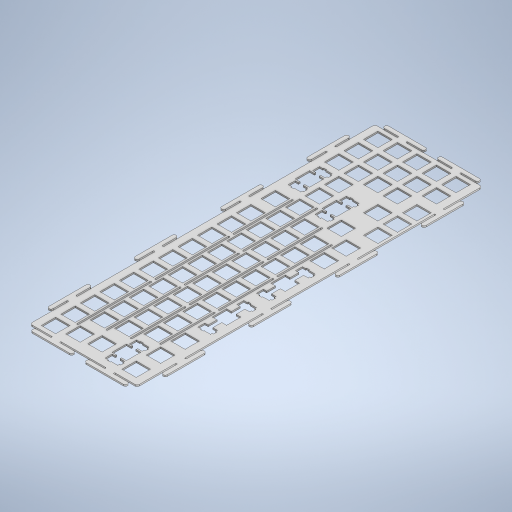
# Autodesk Inventor part: 定位板
Saved by Autodesk Inventor 2024 (Build 280153000, 153)
## iProperties
Created: 2023-06-19
Part Number: 定位板
Material: 常规
Document SubType Name: Modeling
Designer: 24564
Density: 1 g/cm^3
Appearance: 默认
Author: 24564
Autodesk Inventor part; units mm, degrees
(part 1 of 2)
ref_plane "YZ Plane" through (0, 0, 0) normal (1, 0, 0) x (0, 1, 0)
ref_plane "XZ Plane" through (0, 0, 0) normal (0, 1, 0) x (-1, 0, 0)
ref_plane "XY Plane" through (0, 0, 0) normal (0, 0, 1) x (1, 0, 0)
sketch "草图1" plane through (0, 0, 0) normal (0, 1, 0) x (-1, 0, 0)
  line L0 (104.4878, -334.8489) -> (0, -334.8489)
  line L1 (0, 1.4754) -> (104.4878, 1.4754)
  line L2 (16.5254, -235.8869) -> (16.5254, -249.8869)
  line L3 (16.5254, -249.8869) -> (2.5259, -249.8869)
  line L4 (2.5259, -235.8869) -> (16.5254, -235.8869)
  line L5 (16.5254, -254.9369) -> (16.5254, -268.9369)
  line L6 (16.5254, -268.9369) -> (2.5259, -268.9369)
  line L7 (2.5259, -254.9369) -> (16.5254, -254.9369)
  line L8 (16.5254, -273.9869) -> (16.5254, -287.9869)
  line L9 (16.5254, -287.9869) -> (2.5259, -287.9869)
  line L10 (2.5259, -273.9869) -> (16.5254, -273.9869)
  line L11 (21.2879, -93.0121) -> (16.5874, -93.0121)
  line L12 (16.5874, -93.0121) -> (16.5874, -84.3359)
  line L13 (16.5874, -84.3359) -> (19.8176, -84.3359)
  line L14 (19.8176, -84.3359) -> (19.8176, -77.5862)
  line L15 (19.8176, -77.5862) -> (16.5874, -77.5862)
  line L16 (16.5874, -77.5862) -> (16.5874, -76.7607)
  line L17 (16.5874, -76.7607) -> (13.7886, -76.7607)
  line L18 (13.7886, -76.7607) -> (13.7886, -77.5862)
  line L19 (13.7886, -77.5862) -> (7.5186, -77.5862)
  line L20 (7.5186, -77.5862) -> (7.5186, -79.3116)
  line L21 (7.5186, -79.3116) -> (6.3183, -79.3116)
  line L22 (6.3183, -79.3116) -> (6.3183, -82.6119)
  line L23 (6.3183, -82.6119) -> (7.5186, -82.6119)
  line L24 (7.5186, -82.6119) -> (7.5186, -84.3359)
  line L25 (7.5186, -84.3359) -> (11.9889, -84.3359)
  line L26 (11.9889, -84.3359) -> (11.9889, -93.0121)
  line L27 (11.9889, -93.0121) -> (7.2884, -93.0121)
  line L28 (7.2884, -93.0121) -> (7.2884, -107.0119)
  line L29 (7.2884, -107.0119) -> (11.9889, -107.0119)
  line L30 (11.9889, -107.0119) -> (11.9889, -115.6859)
  line L31 (11.9889, -115.6859) -> (7.5186, -115.6859)
  line L32 (7.5186, -115.6859) -> (7.5186, -117.4119)
  line L33 (7.5186, -117.4119) -> (6.3183, -117.4119)
  line L34 (6.3183, -117.4119) -> (6.3183, -120.7119)
  line L35 (6.3183, -120.7119) -> (7.5186, -120.7119)
  line L36 (7.5186, -120.7119) -> (7.5186, -122.4359)
  line L37 (7.5186, -122.4359) -> (13.7886, -122.4359)
  line L38 (13.7886, -122.4359) -> (13.7886, -123.2619)
  line L39 (13.7886, -123.2619) -> (16.5874, -123.2619)
  line L40 (16.5874, -123.2619) -> (16.5874, -122.4359)
  line L41 (16.5874, -122.4359) -> (19.8176, -122.4359)
  line L42 (19.8176, -122.4359) -> (19.8176, -115.6859)
  line L43 (19.8176, -115.6859) -> (16.5874, -115.6859)
  line L44 (16.5874, -115.6859) -> (16.5874, -107.0119)
  line L45 (16.5874, -107.0119) -> (21.2879, -107.0119)
  line L46 (21.2879, -107.0119) -> (21.2879, -93.0121)
  line L47 (21.2879, -150.1619) -> (16.5874, -150.1619)
  line L48 (16.5874, -150.1619) -> (16.5874, -141.4859)
  line L49 (16.5874, -141.4859) -> (19.8176, -141.4859)
  line L50 (19.8176, -141.4859) -> (19.8176, -134.7359)
  line L51 (19.8176, -134.7359) -> (16.5874, -134.7359)
  line L52 (16.5874, -134.7359) -> (16.5874, -133.9109)
  line L53 (16.5874, -133.9109) -> (13.7886, -133.9109)
  line L54 (13.7886, -133.9109) -> (13.7886, -134.7359)
  line L55 (13.7886, -134.7359) -> (7.5186, -134.7359)
  line L56 (7.5186, -134.7359) -> (7.5186, -136.4619)
  line L57 (7.5186, -136.4619) -> (6.3183, -136.4619)
  line L58 (6.3183, -136.4619) -> (6.3183, -139.7619)
  line L59 (6.3183, -139.7619) -> (7.5186, -139.7619)
  line L60 (7.5186, -139.7619) -> (7.5186, -141.4859)
  line L61 (7.5186, -141.4859) -> (11.9889, -141.4859)
  line L62 (11.9889, -141.4859) -> (11.9889, -150.1619)
  line L63 (11.9889, -150.1619) -> (7.2884, -150.1619)
  line L64 (7.2884, -150.1619) -> (7.2884, -164.1619)
  line L65 (7.2884, -164.1619) -> (11.9889, -164.1619)
  line L66 (11.9889, -164.1619) -> (11.9889, -172.8359)
  line L67 (11.9889, -172.8359) -> (7.5186, -172.8359)
  line L68 (7.5186, -172.8359) -> (7.5186, -174.5619)
  line L69 (7.5186, -174.5619) -> (6.3183, -174.5619)
  line L70 (6.3183, -174.5619) -> (6.3183, -177.8619)
  line L71 (6.3183, -177.8619) -> (7.5186, -177.8619)
  line L72 (7.5186, -177.8619) -> (7.5186, -179.5859)
  line L73 (7.5186, -179.5859) -> (13.7886, -179.5859)
  line L74 (13.7886, -179.5859) -> (13.7886, -180.4119)
  line L75 (13.7886, -180.4119) -> (16.5874, -180.4119)
  line L76 (16.5874, -180.4119) -> (16.5874, -179.5859)
  line L77 (16.5874, -179.5859) -> (19.8176, -179.5859)
  line L78 (19.8176, -179.5859) -> (19.8176, -172.8359)
  line L79 (19.8176, -172.8359) -> (16.5874, -172.8359)
  line L80 (16.5874, -172.8359) -> (16.5874, -164.1619)
  line L81 (16.5874, -164.1619) -> (21.2879, -164.1619)
  line L82 (21.2879, -164.1619) -> (21.2879, -150.1619)
  line L83 (21.2879, -4.9058) -> (21.2879, -18.9053)
  line L84 (21.2879, -18.9053) -> (7.2884, -18.9053)
  line L85 (7.2884, -18.9053) -> (7.2884, -4.9058)
  line L86 (7.2884, -4.9058) -> (21.2879, -4.9058)
  line L87 (21.2879, -28.7169) -> (21.2879, -42.7177)
  line L88 (21.2879, -42.7177) -> (7.2884, -42.7177)
  line L89 (7.2884, -42.7177) -> (7.2884, -28.7169)
  line L90 (7.2884, -28.7169) -> (21.2879, -28.7169)
  line L91 (21.2879, -52.5309) -> (21.2879, -66.5302)
  line L92 (21.2879, -66.5302) -> (7.2884, -66.5302)
  line L93 (7.2884, -66.5302) -> (7.2884, -52.5309)
  line L94 (7.2884, -52.5309) -> (21.2879, -52.5309)
  line L95 (21.2879, -188.2619) -> (21.2879, -202.2619)
  line L96 (21.2879, -202.2619) -> (7.2884, -202.2619)
  line L97 (7.2884, -202.2619) -> (7.2884, -188.2619)
  line L98 (7.2884, -188.2619) -> (21.2879, -188.2619)
  line L99 (21.2879, -209.6919) -> (21.2879, -223.6929)
  line L100 (21.2879, -223.6929) -> (7.2884, -223.6929)
  line L101 (7.2884, -223.6929) -> (7.2884, -209.6919)
  line L102 (7.2884, -209.6919) -> (21.2879, -209.6919)
  line L103 (21.2879, -297.7999) -> (21.2879, -311.7989)
  line L104 (21.2879, -311.7989) -> (7.2884, -311.7989)
  line L105 (7.2884, -311.7989) -> (7.2884, -297.7999)
  line L106 (7.2884, -297.7999) -> (21.2879, -297.7999)
  line L107 (21.2879, -316.8499) -> (21.2879, -330.8489)
  line L108 (21.2879, -330.8489) -> (7.2884, -330.8489)
  line L109 (7.2884, -330.8489) -> (7.2884, -316.8499)
  line L110 (7.2884, -316.8499) -> (21.2879, -316.8499)
  line L111 (35.5753, -254.9369) -> (35.5753, -268.9369)
  line L112 (35.5753, -268.9369) -> (21.5759, -268.9369)
  line L113 (21.5759, -268.9369) -> (21.5759, -254.9369)
  line L114 (21.5759, -254.9369) -> (35.5753, -254.9369)
  line L115 (40.3378, -14.4308) -> (35.6374, -14.4308)
  line L116 (35.6374, -14.4308) -> (35.6374, -12.9053)
  line L117 (35.6374, -12.9053) -> (38.8675, -12.9053)
  line L118 (38.8675, -12.9053) -> (38.8675, -6.1557)
  line L119 (38.8675, -6.1557) -> (35.6374, -6.1557)
  line L120 (35.6374, -6.1557) -> (35.6374, -5.3302)
  line L121 (35.6374, -5.3302) -> (32.8386, -5.3302)
  line L122 (32.8386, -5.3302) -> (32.8386, -6.1557)
  line L123 (32.8386, -6.1557) -> (26.5686, -6.1557)
  line L124 (26.5686, -6.1557) -> (26.5686, -7.881)
  line L125 (26.5686, -7.881) -> (25.3683, -7.881)
  line L126 (25.3683, -7.881) -> (25.3683, -11.18)
  line L127 (25.3683, -11.18) -> (26.5686, -11.18)
  line L128 (26.5686, -11.18) -> (26.5686, -12.9053)
  line L129 (26.5686, -12.9053) -> (31.0375, -12.9053)
  line L130 (31.0375, -12.9053) -> (31.0375, -14.4308)
  line L131 (31.0375, -14.4308) -> (26.3384, -14.4308)
  line L132 (26.3384, -14.4308) -> (26.3384, -28.4303)
  line L133 (26.3384, -28.4303) -> (31.0375, -28.4303)
  line L134 (31.0375, -28.4303) -> (31.0375, -29.9558)
  line L135 (31.0375, -29.9558) -> (26.5686, -29.9558)
  line L136 (26.5686, -29.9558) -> (26.5686, -31.6797)
  line L137 (26.5686, -31.6797) -> (25.3683, -31.6797)
  line L138 (25.3683, -31.6797) -> (25.3683, -34.9801)
  line L139 (25.3683, -34.9801) -> (26.5686, -34.9801)
  line L140 (26.5686, -34.9801) -> (26.5686, -36.7053)
  line L141 (26.5686, -36.7053) -> (32.8386, -36.7053)
  line L142 (32.8386, -36.7053) -> (32.8386, -37.5308)
  line L143 (32.8386, -37.5308) -> (35.6374, -37.5308)
  line L144 (35.6374, -37.5308) -> (35.6374, -36.7053)
  line L145 (35.6374, -36.7053) -> (38.8675, -36.7053)
  line L146 (38.8675, -36.7053) -> (38.8675, -29.9558)
  line L147 (38.8675, -29.9558) -> (35.6374, -29.9558)
  line L148 (35.6374, -29.9558) -> (35.6374, -28.4303)
  line L149 (35.6374, -28.4303) -> (40.3378, -28.4303)
  line L150 (40.3378, -28.4303) -> (40.3378, -14.4308)
  line L151 (40.3378, -45.3871) -> (40.3378, -59.3864)
  line L152 (40.3378, -59.3864) -> (26.3384, -59.3864)
  line L153 (26.3384, -59.3864) -> (26.3384, -45.3871)
  line L154 (26.3384, -45.3871) -> (40.3378, -45.3871)
  line L155 (40.3378, -64.4371) -> (40.3378, -78.4364)
  line L156 (40.3378, -78.4364) -> (26.3384, -78.4364)
  line L157 (26.3384, -78.4364) -> (26.3384, -64.4371)
  line L158 (26.3384, -64.4371) -> (40.3378, -64.4371)
  line L159 (40.3378, -83.4871) -> (40.3378, -97.4864)
  line L160 (40.3378, -97.4864) -> (26.3384, -97.4864)
  line L161 (26.3384, -97.4864) -> (26.3384, -83.4871)
  line L162 (26.3384, -83.4871) -> (40.3378, -83.4871)
  line L163 (40.3378, -102.5369) -> (40.3378, -116.5369)
  line L164 (40.3378, -116.5369) -> (26.3384, -116.5369)
  line L165 (26.3384, -116.5369) -> (26.3384, -102.5369)
  line L166 (26.3384, -102.5369) -> (40.3378, -102.5369)
  line L167 (40.3378, -121.5869) -> (40.3378, -135.5869)
  line L168 (40.3378, -135.5869) -> (26.3384, -135.5869)
  line L169 (26.3384, -135.5869) -> (26.3384, -121.5869)
  line L170 (26.3384, -121.5869) -> (40.3378, -121.5869)
  line L171 (40.3378, -140.6369) -> (40.3378, -154.6369)
  line L172 (40.3378, -154.6369) -> (26.3384, -154.6369)
  line L173 (26.3384, -154.6369) -> (26.3384, -140.6369)
  line L174 (26.3384, -140.6369) -> (40.3378, -140.6369)
  line L175 (40.3378, -159.6869) -> (40.3378, -173.6869)
  line L176 (40.3378, -173.6869) -> (26.3384, -173.6869)
  line L177 (26.3384, -173.6869) -> (26.3384, -159.6869)
  line L178 (26.3384, -159.6869) -> (40.3378, -159.6869)
  line L179 (40.3378, -178.7369) -> (40.3378, -192.7369)
  line L180 (40.3378, -192.7369) -> (26.3384, -192.7369)
  line L181 (26.3384, -192.7369) -> (26.3384, -178.7369)
  line L182 (26.3384, -178.7369) -> (40.3378, -178.7369)
  line L183 (40.3378, -197.7869) -> (40.3378, -211.7869)
  line L184 (40.3378, -211.7869) -> (26.3384, -211.7869)
  line L185 (26.3384, -211.7869) -> (26.3384, -197.7869)
  line L186 (26.3384, -197.7869) -> (40.3378, -197.7869)
  line L187 (40.3378, -223.9809) -> (40.3378, -237.9799)
  line L188 (40.3378, -237.9799) -> (26.3384, -237.9799)
  line L189 (26.3384, -237.9799) -> (26.3384, -223.9809)
  line L190 (26.3384, -223.9809) -> (40.3378, -223.9809)
  line L191 (40.3378, -278.7499) -> (40.3378, -292.7489)
  line L192 (40.3378, -292.7489) -> (26.3384, -292.7489)
  line L193 (26.3384, -292.7489) -> (26.3384, -278.7499)
  line L194 (26.3384, -278.7499) -> (40.3378, -278.7499)
  line L195 (40.3378, -297.7999) -> (40.3378, -311.7989)
  line L196 (40.3378, -311.7989) -> (26.3384, -311.7989)
  line L197 (26.3384, -311.7989) -> (26.3384, -297.7999)
  line L198 (26.3384, -297.7999) -> (40.3378, -297.7999)
  line L199 (40.3378, -316.8499) -> (40.3378, -330.8489)
  line L200 (40.3378, -330.8489) -> (26.3384, -330.8489)
  line L201 (26.3384, -330.8489) -> (26.3384, -316.8499)
  line L202 (26.3384, -316.8499) -> (40.3378, -316.8499)
  line L203 (59.3878, -238.2669) -> (54.6874, -238.2669)
  line L204 (54.6874, -238.2669) -> (54.6874, -236.7429)
  line L205 (54.6874, -236.7429) -> (57.9175, -236.7429)
  line L206 (57.9175, -236.7429) -> (57.9175, -229.9919)
  line L207 (57.9175, -229.9919) -> (54.6874, -229.9919)
  line L208 (54.6874, -229.9919) -> (54.6874, -229.1679)
  line L209 (54.6874, -229.1679) -> (51.8885, -229.1679)
  line L210 (51.8885, -229.1679) -> (51.8885, -229.9919)
  line L211 (51.8885, -229.9919) -> (45.6186, -229.9919)
  line L212 (45.6186, -229.9919) -> (45.6186, -231.7169)
  line L213 (45.6186, -231.7169) -> (44.4184, -231.7169)
  line L214 (44.4184, -231.7169) -> (44.4184, -235.0179)
  line L215 (44.4184, -235.0179) -> (45.6186, -235.0179)
  line L216 (45.6186, -235.0179) -> (45.6186, -236.7429)
  line L217 (45.6186, -236.7429) -> (50.0876, -236.7429)
  line L218 (50.0876, -236.7429) -> (50.0876, -238.2669)
  line L219 (50.0876, -238.2669) -> (45.3886, -238.2669)
  line L220 (45.3886, -238.2669) -> (45.3886, -252.2659)
  line L221 (45.3886, -252.2659) -> (50.0876, -252.2659)
  line L222 (50.0876, -252.2659) -> (50.0876, -253.7919)
  line L223 (50.0876, -253.7919) -> (45.6186, -253.7919)
  line L224 (45.6186, -253.7919) -> (45.6186, -255.5159)
  line L225 (45.6186, -255.5159) -> (44.4184, -255.5159)
  line L226 (44.4184, -255.5159) -> (44.4184, -258.8179)
  line L227 (44.4184, -258.8179) -> (45.6186, -258.8179)
  line L228 (45.6186, -258.8179) -> (45.6186, -260.5429)
  line L229 (45.6186, -260.5429) -> (51.8885, -260.5429)
  line L230 (51.8885, -260.5429) -> (51.8885, -261.3669)
  line L231 (51.8885, -261.3669) -> (54.6874, -261.3669)
  line L232 (54.6874, -261.3669) -> (54.6874, -260.5429)
  line L233 (54.6874, -260.5429) -> (57.9175, -260.5429)
  line L234 (57.9175, -260.5429) -> (57.9175, -253.7919)
  line L235 (57.9175, -253.7919) -> (54.6874, -253.7919)
  line L236 (54.6874, -253.7919) -> (54.6874, -252.2659)
  line L237 (54.6874, -252.2659) -> (59.3878, -252.2659)
  line L238 (59.3878, -252.2659) -> (59.3878, -238.2669)
  line L239 (59.3878, -9.6669) -> (59.3878, -23.6678)
  line L240 (59.3878, -23.6678) -> (45.3886, -23.6678)
  line L241 (45.3886, -23.6678) -> (45.3886, -9.6669)
  line L242 (45.3886, -9.6669) -> (59.3878, -9.6669)
  line L243 (59.3878, -35.8621) -> (59.3878, -49.8614)
  line L244 (59.3878, -49.8614) -> (45.3886, -49.8614)
  line L245 (45.3886, -49.8614) -> (45.3886, -35.8621)
  line L246 (45.3886, -35.8621) -> (59.3878, -35.8621)
  line L247 (59.3878, -54.9121) -> (59.3878, -68.9114)
  line L248 (59.3878, -68.9114) -> (45.3886, -68.9114)
  line L249 (45.3886, -68.9114) -> (45.3886, -54.9121)
  line L250 (45.3886, -54.9121) -> (59.3878, -54.9121)
  line L251 (59.3878, -73.9621) -> (59.3878, -87.9614)
  line L252 (59.3878, -87.9614) -> (45.3886, -87.9614)
  line L253 (45.3886, -87.9614) -> (45.3886, -73.9621)
  line L254 (45.3886, -73.9621) -> (59.3878, -73.9621)
  line L255 (59.3878, -93.0121) -> (59.3878, -107.0119)
  line L256 (59.3878, -107.0119) -> (45.3886, -107.0119)
  line L257 (45.3886, -107.0119) -> (45.3886, -93.0121)
  line L258 (45.3886, -93.0121) -> (59.3878, -93.0121)
  line L259 (59.3878, -112.0619) -> (59.3878, -126.0619)
  line L260 (59.3878, -126.0619) -> (45.3886, -126.0619)
  line L261 (45.3886, -126.0619) -> (45.3886, -112.0619)
  line L262 (45.3886, -112.0619) -> (59.3878, -112.0619)
  line L263 (59.3878, -131.1119) -> (59.3878, -145.1119)
  line L264 (59.3878, -145.1119) -> (45.3886, -145.1119)
  line L265 (45.3886, -145.1119) -> (45.3886, -131.1119)
  line L266 (45.3886, -131.1119) -> (59.3878, -131.1119)
  line L267 (59.3878, -150.1619) -> (59.3878, -164.1619)
  line L268 (59.3878, -164.1619) -> (45.3886, -164.1619)
  line L269 (45.3886, -164.1619) -> (45.3886, -150.1619)
  line L270 (45.3886, -150.1619) -> (59.3878, -150.1619)
  line L271 (59.3878, -169.2119) -> (59.3878, -183.2119)
  line L272 (59.3878, -183.2119) -> (45.3886, -183.2119)
  line L273 (45.3886, -183.2119) -> (45.3886, -169.2119)
  line L274 (45.3886, -169.2119) -> (59.3878, -169.2119)
  line L275 (59.3878, -188.2619) -> (59.3878, -202.2619)
  line L276 (59.3878, -202.2619) -> (45.3886, -202.2619)
  line L277 (45.3886, -202.2619) -> (45.3886, -188.2619)
  line L278 (45.3886, -188.2619) -> (59.3878, -188.2619)
  line L279 (59.3878, -207.3119) -> (59.3878, -221.3119)
  line L280 (59.3878, -221.3119) -> (45.3886, -221.3119)
  line L281 (45.3886, -221.3119) -> (45.3886, -207.3119)
  line L282 (45.3886, -207.3119) -> (59.3878, -207.3119)
  line L283 (59.3878, -278.7499) -> (59.3878, -292.7489)
  line L284 (59.3878, -292.7489) -> (45.3886, -292.7489)
  line L285 (45.3886, -292.7489) -> (45.3886, -278.7499)
  line L286 (45.3886, -278.7499) -> (59.3878, -278.7499)
  line L287 (59.3878, -297.7999) -> (59.3878, -311.7989)
  line L288 (59.3878, -311.7989) -> (45.3886, -311.7989)
  line L289 (45.3886, -311.7989) -> (45.3886, -297.7999)
  line L290 (45.3886, -297.7999) -> (59.3878, -297.7999)
  line L291 (59.3878, -316.8499) -> (59.3878, -330.8489)
  line L292 (59.3878, -330.8489) -> (45.3886, -330.8489)
  line L293 (45.3886, -330.8489) -> (45.3886, -316.8499)
  line L294 (45.3886, -316.8499) -> (59.3878, -316.8499)
  line L295 (78.4378, -7.2871) -> (78.4378, -21.2866)
  line L296 (78.4378, -21.2866) -> (64.4386, -21.2866)
  line L297 (64.4386, -21.2866) -> (64.4386, -7.2871)
  line L298 (64.4386, -7.2871) -> (78.4378, -7.2871)
  line L299 (78.4378, -31.0996) -> (78.4378, -45.0989)
  line L300 (78.4378, -45.0989) -> (64.4386, -45.0989)
  line L301 (64.4386, -45.0989) -> (64.4386, -31.0996)
  line L302 (64.4386, -31.0996) -> (78.4378, -31.0996)
  line L303 (78.4378, -50.1496) -> (78.4378, -64.1489)
  line L304 (78.4378, -64.1489) -> (64.4386, -64.1489)
  line L305 (64.4386, -64.1489) -> (64.4386, -50.1496)
  line L306 (64.4386, -50.1496) -> (78.4378, -50.1496)
  line L307 (78.4378, -69.1996) -> (78.4378, -83.1989)
  line L308 (78.4378, -83.1989) -> (64.4386, -83.1989)
  line L309 (64.4386, -83.1989) -> (64.4386, -69.1996)
  line L310 (64.4386, -69.1996) -> (78.4378, -69.1996)
  line L311 (78.4378, -88.2496) -> (78.4378, -102.2489)
  line L312 (78.4378, -102.2489) -> (64.4386, -102.2489)
  line L313 (64.4386, -102.2489) -> (64.4386, -88.2496)
  line L314 (64.4386, -88.2496) -> (78.4378, -88.2496)
  line L315 (78.4378, -107.2999) -> (78.4378, -121.2989)
  line L316 (78.4378, -121.2989) -> (64.4386, -121.2989)
  line L317 (64.4386, -121.2989) -> (64.4386, -107.2999)
  line L318 (64.4386, -107.2999) -> (78.4378, -107.2999)
  line L319 (78.4378, -126.3499) -> (78.4378, -140.3489)
  line L320 (78.4378, -140.3489) -> (64.4386, -140.3489)
  line L321 (64.4386, -140.3489) -> (64.4386, -126.3499)
  line L322 (64.4386, -126.3499) -> (78.4378, -126.3499)
  line L323 (78.4378, -145.3999) -> (78.4378, -159.3989)
  line L324 (78.4378, -159.3989) -> (64.4386, -159.3989)
  line L325 (64.4386, -159.3989) -> (64.4386, -145.3999)
  line L326 (64.4386, -145.3999) -> (78.4378, -145.3999)
  line L327 (78.4378, -164.4499) -> (78.4378, -178.4489)
  line L328 (78.4378, -178.4489) -> (64.4386, -178.4489)
  line L329 (64.4386, -178.4489) -> (64.4386, -164.4499)
  line L330 (64.4386, -164.4499) -> (78.4378, -164.4499)
  line L331 (78.4378, -183.4999) -> (78.4378, -197.4989)
  line L332 (78.4378, -197.4989) -> (64.4386, -197.4989)
  line L333 (64.4386, -197.4989) -> (64.4386, -183.4999)
  line L334 (64.4386, -183.4999) -> (78.4378, -183.4999)
  line L335 (78.4378, -202.5499) -> (78.4378, -216.5489)
  line L336 (78.4378, -216.5489) -> (64.4386, -216.5489)
  line L337 (64.4386, -216.5489) -> (64.4386, -202.5499)
  line L338 (64.4386, -202.5499) -> (78.4378, -202.5499)
  line L339 (78.4378, -221.5999) -> (78.4378, -235.5989)
  line L340 (78.4378, -235.5989) -> (64.4386, -235.5989)
  line L341 (64.4386, -235.5989) -> (64.4386, -221.5999)
  line L342 (64.4386, -221.5999) -> (78.4378, -221.5999)
  line L343 (78.4378, -240.6499) -> (78.4378, -254.6489)
  line L344 (78.4378, -254.6489) -> (64.4386, -254.6489)
  line L345 (64.4386, -254.6489) -> (64.4386, -240.6499)
  line L346 (64.4386, -240.6499) -> (78.4378, -240.6499)
  line L347 (78.4378, -259.6999) -> (78.4378, -273.6989)
  line L348 (78.4378, -273.6989) -> (64.4386, -273.6989)
  line L349 (64.4386, -273.6989) -> (64.4386, -259.6999)
  line L350 (64.4386, -259.6999) -> (78.4378, -259.6999)
  line L351 (78.4378, -278.7499) -> (78.4378, -292.7489)
  line L352 (78.4378, -292.7489) -> (64.4386, -292.7489)
  line L353 (64.4386, -292.7489) -> (64.4386, -278.7499)
  line L354 (64.4386, -278.7499) -> (78.4378, -278.7499)
  line L355 (78.4378, -297.7999) -> (78.4378, -311.7989)
  line L356 (78.4378, -311.7989) -> (64.4386, -311.7989)
  line L357 (64.4386, -311.7989) -> (64.4386, -297.7999)
  line L358 (64.4386, -297.7999) -> (78.4378, -297.7999)
  line L359 (78.4378, -316.8499) -> (78.4378, -330.8489)
  line L360 (78.4378, -330.8489) -> (64.4386, -330.8489)
  line L361 (64.4386, -330.8489) -> (64.4386, -316.8499)
  line L362 (64.4386, -316.8499) -> (78.4378, -316.8499)
  line L363 (97.4878, -250.1749) -> (92.7874, -250.1749)
  line L364 (92.7874, -250.1749) -> (92.7874, -248.6489)
  line L365 (92.7874, -248.6489) -> (96.0175, -248.6489)
  line L366 (96.0175, -248.6489) -> (96.0175, -241.8999)
  line L367 (96.0175, -241.8999) -> (92.7874, -241.8999)
  line L368 (92.7874, -241.8999) -> (92.7874, -241.0739)
  line L369 (92.7874, -241.0739) -> (89.9885, -241.0739)
  line L370 (89.9885, -241.0739) -> (89.9885, -241.8999)
  line L371 (89.9885, -241.8999) -> (83.7186, -241.8999)
  line L372 (83.7186, -241.8999) -> (83.7186, -243.6249)
  line L373 (83.7186, -243.6249) -> (82.5184, -243.6249)
  line L374 (82.5184, -243.6249) -> (82.5184, -246.9239)
  line L375 (82.5184, -246.9239) -> (83.7186, -246.9239)
  line L376 (83.7186, -246.9239) -> (83.7186, -248.6489)
  line L377 (83.7186, -248.6489) -> (88.1876, -248.6489)
  line L378 (88.1876, -248.6489) -> (88.1876, -250.1749)
  line L379 (88.1876, -250.1749) -> (83.4886, -250.1749)
  line L380 (83.4886, -250.1749) -> (83.4886, -264.1739)
  line L381 (83.4886, -264.1739) -> (88.1876, -264.1739)
  line L382 (88.1876, -264.1739) -> (88.1876, -265.6999)
  line L383 (88.1876, -265.6999) -> (83.7186, -265.6999)
  line L384 (83.7186, -265.6999) -> (83.7186, -267.4249)
  line L385 (83.7186, -267.4249) -> (82.5184, -267.4249)
  line L386 (82.5184, -267.4249) -> (82.5184, -270.7239)
  line L387 (82.5184, -270.7239) -> (83.7186, -270.7239)
  line L388 (83.7186, -270.7239) -> (83.7186, -272.4489)
  line L389 (83.7186, -272.4489) -> (89.9885, -272.4489)
  line L390 (89.9885, -272.4489) -> (89.9885, -273.2749)
  line L391 (89.9885, -273.2749) -> (92.7874, -273.2749)
  line L392 (92.7874, -273.2749) -> (92.7874, -272.4489)
  line L393 (92.7874, -272.4489) -> (96.0175, -272.4489)
  line L394 (96.0175, -272.4489) -> (96.0175, -265.6999)
  line L395 (96.0175, -265.6999) -> (92.7874, -265.6999)
  line L396 (92.7874, -265.6999) -> (92.7874, -264.1739)
  line L397 (92.7874, -264.1739) -> (97.4878, -264.1739)
  line L398 (97.4878, -264.1739) -> (97.4878, -250.1749)
  line L399 (97.4878, -2.5246) -> (97.4878, -16.5241)
  line L400 (97.4878, -16.5241) -> (83.4886, -16.5241)
  line L401 (83.4886, -16.5241) -> (83.4886, -2.5246)
  line L402 (83.4886, -2.5246) -> (97.4878, -2.5246)
  line L403 (97.4878, -21.5746) -> (97.4878, -35.5739)
  line L404 (97.4878, -35.5739) -> (83.4886, -35.5739)
  line L405 (83.4886, -35.5739) -> (83.4886, -21.5746)
  line L406 (83.4886, -21.5746) -> (97.4878, -21.5746)
  line L407 (97.4878, -40.6246) -> (97.4878, -54.6239)
  line L408 (97.4878, -54.6239) -> (83.4886, -54.6239)
  line L409 (83.4886, -54.6239) -> (83.4886, -40.6246)
  line L410 (83.4886, -40.6246) -> (97.4878, -40.6246)
  line L411 (97.4878, -59.6746) -> (97.4878, -73.6739)
  line L412 (97.4878, -73.6739) -> (83.4886, -73.6739)
  line L413 (83.4886, -73.6739) -> (83.4886, -59.6746)
  line L414 (83.4886, -59.6746) -> (97.4878, -59.6746)
  line L415 (97.4878, -78.7246) -> (97.4878, -92.7239)
  line L416 (97.4878, -92.7239) -> (83.4886, -92.7239)
  line L417 (83.4886, -92.7239) -> (83.4886, -78.7246)
  line L418 (83.4886, -78.7246) -> (97.4878, -78.7246)
  line L419 (97.4878, -97.7732) -> (97.4878, -111.7739)
  line L420 (97.4878, -111.7739) -> (83.4886, -111.7739)
  line L421 (83.4886, -111.7739) -> (83.4886, -97.7732)
  line L422 (83.4886, -97.7732) -> (97.4878, -97.7732)
  line L423 (97.4878, -116.8229) -> (97.4878, -130.8239)
  line L424 (97.4878, -130.8239) -> (83.4886, -130.8239)
  line L425 (83.4886, -130.8239) -> (83.4886, -116.8229)
  line L426 (83.4886, -116.8229) -> (97.4878, -116.8229)
  line L427 (97.4878, -135.8749) -> (97.4878, -149.8739)
  line L428 (97.4878, -149.8739) -> (83.4886, -149.8739)
  line L429 (83.4886, -149.8739) -> (83.4886, -135.8749)
  line L430 (83.4886, -135.8749) -> (97.4878, -135.8749)
  line L431 (97.4878, -154.9249) -> (97.4878, -168.9239)
  line L432 (97.4878, -168.9239) -> (83.4886, -168.9239)
  line L433 (83.4886, -168.9239) -> (83.4886, -154.9249)
  line L434 (83.4886, -154.9249) -> (97.4878, -154.9249)
  line L435 (97.4878, -173.9749) -> (97.4878, -187.9739)
  line L436 (97.4878, -187.9739) -> (83.4886, -187.9739)
  line L437 (83.4886, -187.9739) -> (83.4886, -173.9749)
  line L438 (83.4886, -173.9749) -> (97.4878, -173.9749)
  line L439 (97.4878, -193.0249) -> (97.4878, -207.0239)
  line L440 (97.4878, -207.0239) -> (83.4886, -207.0239)
  line L441 (83.4886, -207.0239) -> (83.4886, -193.0249)
  line L442 (83.4886, -193.0249) -> (97.4878, -193.0249)
  line L443 (97.4878, -216.8369) -> (97.4878, -230.8369)
  line L444 (97.4878, -230.8369) -> (83.4886, -230.8369)
  line L445 (83.4886, -230.8369) -> (83.4886, -216.8369)
  line L446 (83.4886, -216.8369) -> (97.4878, -216.8369)
  line L447 (97.4878, -278.7499) -> (97.4878, -292.7489)
  line L448 (97.4878, -292.7489) -> (83.4886, -292.7489)
  line L449 (83.4886, -292.7489) -> (83.4886, -278.7499)
  line L450 (83.4886, -278.7499) -> (97.4878, -278.7499)
  line L451 (97.4878, -297.7999) -> (97.4878, -311.7989)
  line L452 (97.4878, -311.7989) -> (83.4886, -311.7989)
  line L453 (83.4886, -311.7989) -> (83.4886, -297.7999)
  line L454 (83.4886, -297.7999) -> (97.4878, -297.7999)
  line L455 (97.4878, -316.8499) -> (97.4878, -330.8489)
  line L456 (97.4878, -330.8489) -> (83.4886, -330.8489)
  line L457 (83.4886, -330.8489) -> (83.4886, -316.8499)
  line L458 (83.4886, -316.8499) -> (97.4878, -316.8499)
  line L459 (81.7132, -21.5746) -> (81.7132, -92.7239)
  line L460 (80.2132, -92.7239) -> (80.2132, -21.5746)
  arc A0 (81.7132, -21.5746) -> (80.2132, -21.5746) centre (80.9632, -21.5746) ccw
  arc A1 (80.2132, -92.7239) -> (81.7132, -92.7239) centre (80.9632, -92.7239) ccw
  line L461 (62.6632, -31.0996) -> (62.6632, -102.2489)
  line L462 (61.1632, -102.2489) -> (61.1632, -31.0996)
  arc A2 (62.6632, -31.0996) -> (61.1632, -31.0996) centre (61.9132, -31.0996) ccw
  arc A3 (61.1632, -102.2489) -> (62.6632, -102.2489) centre (61.9132, -102.2489) ccw
  line L463 (62.6632, -107.2999) -> (62.6632, -159.3989)
  line L464 (61.1632, -159.3989) -> (61.1632, -107.2999)
  arc A4 (62.6632, -107.2999) -> (61.1632, -107.2999) centre (61.9132, -107.2999) ccw
  arc A5 (61.1632, -159.3989) -> (62.6632, -159.3989) centre (61.9132, -159.3989) ccw
  line L465 (43.6132, -35.8621) -> (43.6132, -87.9611)
  line L466 (42.1132, -87.9611) -> (42.1132, -35.8621)
  arc A6 (43.6132, -35.8621) -> (42.1132, -35.8621) centre (42.8632, -35.8621) ccw
  arc A7 (42.1132, -87.9611) -> (43.6132, -87.9611) centre (42.8632, -87.9611) ccw
  line L467 (24.5632, -45.3871) -> (24.5632, -97.4861)
  line L468 (23.0632, -97.4861) -> (23.0632, -45.3871)
  arc A8 (24.5632, -45.3871) -> (23.0632, -45.3871) centre (23.8132, -45.3871) ccw
  arc A9 (23.0632, -97.4861) -> (24.5632, -97.4861) centre (23.8132, -97.4861) ccw
  line L469 (24.5632, -102.5369) -> (24.5632, -154.6359)
  line L470 (23.0632, -154.6359) -> (23.0632, -102.5369)
  arc A10 (24.5632, -102.5369) -> (23.0632, -102.5369) centre (23.8132, -102.5369) ccw
  arc A11 (23.0632, -154.6359) -> (24.5632, -154.6359) centre (23.8132, -154.6359) ccw
  line L471 (24.5632, -159.6869) -> (24.5632, -211.7859)
  line L472 (23.0632, -211.7859) -> (23.0632, -159.6869)
  arc A12 (24.5632, -159.6869) -> (23.0632, -159.6869) centre (23.8132, -159.6869) ccw
  arc A13 (23.0632, -211.7859) -> (24.5632, -211.7859) centre (23.8132, -211.7859) ccw
  line L473 (43.6132, -169.2119) -> (43.6132, -221.3109)
  line L474 (42.1132, -221.3109) -> (42.1132, -169.2119)
  arc A14 (43.6132, -169.2119) -> (42.1132, -169.2119) centre (42.8632, -169.2119) ccw
  arc A15 (42.1132, -221.3109) -> (43.6132, -221.3109) centre (42.8632, -221.3109) ccw
  line L475 (43.6132, -93.0121) -> (43.6132, -164.1614)
  line L476 (42.1132, -164.1614) -> (42.1132, -93.0121)
  arc A16 (43.6132, -93.0121) -> (42.1132, -93.0121) centre (42.8632, -93.0121) ccw
  arc A17 (42.1132, -164.1614) -> (43.6132, -164.1614) centre (42.8632, -164.1614) ccw
  line L477 (62.6632, -164.4499) -> (62.6632, -235.5992)
  line L478 (61.1632, -235.5992) -> (61.1632, -164.4499)
  arc A18 (62.6632, -164.4499) -> (61.1632, -164.4499) centre (61.9132, -164.4499) ccw
  arc A19 (61.1632, -235.5992) -> (62.6632, -235.5992) centre (61.9132, -235.5992) ccw
  line L479 (81.7132, -97.7732) -> (81.7132, -168.9225)
  line L480 (80.2132, -168.9225) -> (80.2132, -97.7732)
  arc A20 (81.7132, -97.7732) -> (80.2132, -97.7732) centre (80.9632, -97.7732) ccw
  arc A21 (80.2132, -168.9225) -> (81.7132, -168.9225) centre (80.9632, -168.9225) ccw
  line L481 (81.7132, -173.9749) -> (81.7132, -230.8369)
  line L482 (80.2132, -230.8369) -> (80.2132, -173.9749)
  arc A22 (81.7132, -173.9749) -> (80.2132, -173.9749) centre (80.9632, -173.9749) ccw
  arc A23 (80.2132, -230.8369) -> (81.7132, -230.8369) centre (80.9632, -230.8369) ccw
  line L483 (107.9878, -312.8489) -> (107.9878, -312.8489)
  line L484 (107.9878, -272.8489) -> (107.9878, -272.8489)
  line L485 (109.9878, -274.8489) -> (109.9878, -310.8489)
  line L486 (105.2378, -296.8489) -> (105.2378, -296.8489)
  line L487 (105.2378, -288.8489) -> (105.2378, -288.8489)
  line L488 (105.9878, -310.8489) -> (105.9878, -297.5989)
  line L489 (105.9878, -288.0989) -> (105.9878, -274.8489)
  line L490 (104.4878, -292.8489) -> (109.9878, -292.8489) construction
  arc A24 (105.9878, -297.5989) -> (105.2378, -296.8489) centre (105.2378, -297.5989) ccw
  line L491 (104.4878, -292.8489) -> (104.4878, -334.8489)
  arc A25 (105.2378, -296.8489) -> (104.4878, -297.5989) centre (105.2378, -297.5989) ccw
  arc A26 (105.2378, -288.8489) -> (105.9878, -288.0989) centre (105.2378, -288.0989) ccw
  arc A27 (104.4878, -288.0989) -> (105.2378, -288.8489) centre (105.2378, -288.0989) ccw
  arc A28 (107.9878, -312.8489) -> (109.9878, -310.8489) centre (107.9878, -310.8489) ccw
  arc A29 (105.9878, -310.8489) -> (107.9878, -312.8489) centre (107.9878, -310.8489) ccw
  arc A30 (109.9878, -274.8489) -> (107.9878, -272.8489) centre (107.9878, -274.8489) ccw
  arc A31 (107.9878, -272.8489) -> (105.9878, -274.8489) centre (107.9878, -274.8489) ccw
  line L492 (104.4878, -297.5989) -> (104.4878, -288.0989) construction
  line L493 (0, -334.8489) -> (0, 1.4754)
  line L494 (107.9878, -228.8489) -> (107.9878, -228.8489)
  line L495 (107.9878, -188.8489) -> (107.9878, -188.8489)
  line L496 (109.9878, -190.8489) -> (109.9878, -226.8489)
  line L497 (105.2378, -212.8489) -> (105.2378, -212.8489)
  line L498 (105.2378, -204.8489) -> (105.2378, -204.8489)
  line L499 (105.9878, -226.8489) -> (105.9878, -213.5989)
  line L500 (105.9878, -204.0989) -> (105.9878, -190.8489)
  line L501 (104.4878, -208.8489) -> (109.9878, -208.8489) construction
  arc A32 (105.9878, -213.5989) -> (105.2378, -212.8489) centre (105.2378, -213.5989) ccw
  arc A33 (105.2378, -212.8489) -> (104.4878, -213.5989) centre (105.2378, -213.5989) ccw
  arc A34 (105.2378, -204.8489) -> (105.9878, -204.0989) centre (105.2378, -204.0989) ccw
  arc A35 (104.4878, -204.0989) -> (105.2378, -204.8489) centre (105.2378, -204.0989) ccw
  arc A36 (107.9878, -228.8489) -> (109.9878, -226.8489) centre (107.9878, -226.8489) ccw
  arc A37 (105.9878, -226.8489) -> (107.9878, -228.8489) centre (107.9878, -226.8489) ccw
  arc A38 (109.9878, -190.8489) -> (107.9878, -188.8489) centre (107.9878, -190.8489) ccw
  arc A39 (107.9878, -188.8489) -> (105.9878, -190.8489) centre (107.9878, -190.8489) ccw
  line L502 (104.4878, -213.5989) -> (104.4878, -204.0989) construction
  line L503 (107.9878, -144.5246) -> (107.9878, -144.5246)
  line L504 (107.9878, -104.5246) -> (107.9878, -104.5246)
  line L505 (109.9878, -106.5246) -> (109.9878, -142.5246)
  line L506 (105.2378, -128.5246) -> (105.2378, -128.5246)
  line L507 (105.2378, -120.5246) -> (105.2378, -120.5246)
  line L508 (105.9878, -142.5246) -> (105.9878, -129.2746)
  line L509 (105.9878, -119.7746) -> (105.9878, -106.5246)
  line L510 (104.4878, -124.5246) -> (109.9878, -124.5246) construction
  arc A40 (105.9878, -129.2746) -> (105.2378, -128.5246) centre (105.2378, -129.2746) ccw
  arc A41 (105.2378, -128.5246) -> (104.4878, -129.2746) centre (105.2378, -129.2746) ccw
  arc A42 (105.2378, -120.5246) -> (105.9878, -119.7746) centre (105.2378, -119.7746) ccw
  arc A43 (104.4878, -119.7746) -> (105.2378, -120.5246) centre (105.2378, -119.7746) ccw
  arc A44 (107.9878, -144.5246) -> (109.9878, -142.5246) centre (107.9878, -142.5246) ccw
  arc A45 (105.9878, -142.5246) -> (107.9878, -144.5246) centre (107.9878, -142.5246) ccw
  arc A46 (109.9878, -106.5246) -> (107.9878, -104.5246) centre (107.9878, -106.5246) ccw
  arc A47 (107.9878, -104.5246) -> (105.9878, -106.5246) centre (107.9878, -106.5246) ccw
  line L511 (104.4878, -129.2746) -> (104.4878, -119.7746) construction
  line L512 (107.9878, -60.5246) -> (107.9878, -60.5246)
  line L513 (107.9878, -20.5246) -> (107.9878, -20.5246)
  line L514 (109.9878, -22.5246) -> (109.9878, -58.5246)
  line L515 (105.2378, -44.5246) -> (105.2378, -44.5246)
  line L516 (105.2378, -36.5246) -> (105.2378, -36.5246)
  line L517 (105.9878, -58.5246) -> (105.9878, -45.2746)
  line L518 (105.9878, -35.7746) -> (105.9878, -22.5246)
  line L519 (104.4878, -40.5246) -> (109.9878, -40.5246) construction
  arc A48 (105.9878, -45.2746) -> (105.2378, -44.5246) centre (105.2378, -45.2746) ccw
  arc A49 (105.2378, -44.5246) -> (104.4878, -45.2746) centre (105.2378, -45.2746) ccw
  arc A50 (105.2378, -36.5246) -> (105.9878, -35.7746) centre (105.2378, -35.7746) ccw
  arc A51 (104.4878, -35.7746) -> (105.2378, -36.5246) centre (105.2378, -35.7746) ccw
  arc A52 (107.9878, -60.5246) -> (109.9878, -58.5246) centre (107.9878, -58.5246) ccw
  arc A53 (105.9878, -58.5246) -> (107.9878, -60.5246) centre (107.9878, -58.5246) ccw
  arc A54 (109.9878, -22.5246) -> (107.9878, -20.5246) centre (107.9878, -22.5246) ccw
  arc A55 (107.9878, -20.5246) -> (105.9878, -22.5246) centre (107.9878, -22.5246) ccw
  line L520 (104.4878, -45.2746) -> (104.4878, -35.7746) construction
  line L521 (104.4878, -208.8489) -> (104.4878, -292.8489)
  line L522 (104.4878, -124.5246) -> (104.4878, -208.8489)
  line L523 (104.4878, 1.4754) -> (104.4878, -40.5246)
  line L524 (104.4878, -40.5246) -> (104.4878, -124.5246)
  line L525 (2.5259, -287.9869) -> (2.5259, -273.9869)
  line L526 (2.5259, -268.9369) -> (2.5259, -254.9369)
  line L527 (2.5259, -249.8869) -> (2.5259, -235.8869)
  line L528 (-0.75, -288.8489) -> (-0.75, -288.8489)
  arc A56 (-0.75, -288.8489) -> (0, -288.0989) centre (-0.75, -288.0989) ccw
  arc A57 (-3.5, -272.8489) -> (-5.5, -274.8489) centre (-3.5, -274.8489) ccw
  line L529 (0, -288.0989) -> (0, -297.5989) construction
  line L530 (-1.5, -274.8489) -> (-1.5, -288.0989)
  arc A58 (-1.5, -288.0989) -> (-0.75, -288.8489) centre (-0.75, -288.0989) ccw
  line L531 (-3.5, -272.8489) -> (-3.5, -272.8489)
  arc A59 (-1.5, -274.8489) -> (-3.5, -272.8489) centre (-3.5, -274.8489) ccw
  line L532 (-5.5, -310.8489) -> (-5.5, -274.8489)
  arc A60 (0, -297.5989) -> (-0.75, -296.8489) centre (-0.75, -297.5989) ccw
  line L533 (-1.5, -297.5989) -> (-1.5, -310.8489)
  arc A61 (-0.75, -296.8489) -> (-1.5, -297.5989) centre (-0.75, -297.5989) ccw
  line L534 (-3.5, -312.8489) -> (-3.5, -312.8489)
  arc A62 (-3.5, -312.8489) -> (-1.5, -310.8489) centre (-3.5, -310.8489) ccw
  line L535 (-0.75, -296.8489) -> (-0.75, -296.8489)
  line L536 (0, -292.8489) -> (-5.5, -292.8489) construction
  arc A63 (-5.5, -310.8489) -> (-3.5, -312.8489) centre (-3.5, -310.8489) ccw
  line L537 (-1.5, -213.5989) -> (-1.5, -226.8489)
  line L538 (-3.5, -228.8489) -> (-3.5, -228.8489)
  arc A64 (-3.5, -228.8489) -> (-1.5, -226.8489) centre (-3.5, -226.8489) ccw
  arc A65 (-5.5, -226.8489) -> (-3.5, -228.8489) centre (-3.5, -226.8489) ccw
  arc A66 (-1.5, -204.0989) -> (-0.75, -204.8489) centre (-0.75, -204.0989) ccw
  arc A67 (-0.75, -204.8489) -> (0, -204.0989) centre (-0.75, -204.0989) ccw
  line L539 (0, -208.8489) -> (-5.5, -208.8489) construction
  line L540 (0, -204.0989) -> (0, -213.5989) construction
  arc A68 (-0.75, -212.8489) -> (-1.5, -213.5989) centre (-0.75, -213.5989) ccw
  arc A69 (0, -213.5989) -> (-0.75, -212.8489) centre (-0.75, -213.5989) ccw
  line L541 (-0.75, -212.8489) -> (-0.75, -212.8489)
  line L542 (-5.5, -226.8489) -> (-5.5, -190.8489)
  line L543 (-1.5, -190.8489) -> (-1.5, -204.0989)
  line L544 (-3.5, -188.8489) -> (-3.5, -188.8489)
  arc A70 (-3.5, -188.8489) -> (-5.5, -190.8489) centre (-3.5, -190.8489) ccw
  arc A71 (-1.5, -190.8489) -> (-3.5, -188.8489) centre (-3.5, -190.8489) ccw
  line L545 (-0.75, -204.8489) -> (-0.75, -204.8489)
  line L546 (-1.5, -129.2746) -> (-1.5, -142.5246)
  line L547 (-3.5, -144.5246) -> (-3.5, -144.5246)
  arc A72 (-3.5, -144.5246) -> (-1.5, -142.5246) centre (-3.5, -142.5246) ccw
  arc A73 (-5.5, -142.5246) -> (-3.5, -144.5246) centre (-3.5, -142.5246) ccw
  arc A74 (-1.5, -119.7746) -> (-0.75, -120.5246) centre (-0.75, -119.7746) ccw
  arc A75 (-0.75, -120.5246) -> (0, -119.7746) centre (-0.75, -119.7746) ccw
  line L548 (0, -124.5246) -> (-5.5, -124.5246) construction
  line L549 (0, -119.7746) -> (0, -129.2746) construction
  arc A76 (-0.75, -128.5246) -> (-1.5, -129.2746) centre (-0.75, -129.2746) ccw
  arc A77 (0, -129.2746) -> (-0.75, -128.5246) centre (-0.75, -129.2746) ccw
  line L550 (-0.75, -128.5246) -> (-0.75, -128.5246)
  line L551 (-5.5, -142.5246) -> (-5.5, -106.5246)
  line L552 (-1.5, -106.5246) -> (-1.5, -119.7746)
  line L553 (-3.5, -104.5246) -> (-3.5, -104.5246)
  arc A78 (-3.5, -104.5246) -> (-5.5, -106.5246) centre (-3.5, -106.5246) ccw
  arc A79 (-1.5, -106.5246) -> (-3.5, -104.5246) centre (-3.5, -106.5246) ccw
  line L554 (-0.75, -120.5246) -> (-0.75, -120.5246)
  line L555 (-1.5, -45.2746) -> (-1.5, -58.5246)
  line L556 (-3.5, -60.5246) -> (-3.5, -60.5246)
  arc A80 (-3.5, -60.5246) -> (-1.5, -58.5246) centre (-3.5, -58.5246) ccw
  arc A81 (-5.5, -58.5246) -> (-3.5, -60.5246) centre (-3.5, -58.5246) ccw
  arc A82 (-1.5, -35.7746) -> (-0.75, -36.5246) centre (-0.75, -35.7746) ccw
  arc A83 (-0.75, -36.5246) -> (0, -35.7746) centre (-0.75, -35.7746) ccw
  line L557 (0, -40.5246) -> (-5.5, -40.5246) construction
  line L558 (0, -35.7746) -> (0, -45.2746) construction
  arc A84 (-0.75, -44.5246) -> (-1.5, -45.2746) centre (-0.75, -45.2746) ccw
  arc A85 (0, -45.2746) -> (-0.75, -44.5246) centre (-0.75, -45.2746) ccw
  line L559 (-0.75, -44.5246) -> (-0.75, -44.5246)
  line L560 (-5.5, -58.5246) -> (-5.5, -22.5246)
  line L561 (-1.5, -22.5246) -> (-1.5, -35.7746)
  line L562 (-3.5, -20.5246) -> (-3.5, -20.5246)
  arc A86 (-3.5, -20.5246) -> (-5.5, -22.5246) centre (-3.5, -22.5246) ccw
  arc A87 (-1.5, -22.5246) -> (-3.5, -20.5246) centre (-3.5, -22.5246) ccw
  line L563 (-0.75, -36.5246) -> (-0.75, -36.5246)
  line L564 (82.4878, 2.2254) -> (82.4878, 2.2254)
  arc A88 (82.4878, 2.2254) -> (83.2378, 1.4754) centre (83.2378, 2.2254) ccw
  arc A89 (98.4878, 4.9754) -> (96.4878, 6.9754) centre (96.4878, 4.9754) ccw
  line L565 (83.2378, 1.4754) -> (73.7378, 1.4754) construction
  line L566 (96.4878, 2.9754) -> (83.2378, 2.9754)
  arc A90 (83.2378, 2.9754) -> (82.4878, 2.2254) centre (83.2378, 2.2254) ccw
  line L567 (98.4878, 4.9754) -> (98.4878, 4.9754)
  arc A91 (96.4878, 2.9754) -> (98.4878, 4.9754) centre (96.4878, 4.9754) ccw
  line L568 (60.4878, 6.9754) -> (96.4878, 6.9754)
  arc A92 (73.7378, 1.4754) -> (74.4878, 2.2254) centre (73.7378, 2.2254) ccw
  line L569 (73.7378, 2.9754) -> (60.4878, 2.9754)
  arc A93 (74.4878, 2.2254) -> (73.7378, 2.9754) centre (73.7378, 2.2254) ccw
  line L570 (58.4878, 4.9754) -> (58.4878, 4.9754)
  arc A94 (58.4878, 4.9754) -> (60.4878, 2.9754) centre (60.4878, 4.9754) ccw
  line L571 (74.4878, 2.2254) -> (74.4878, 2.2254)
  line L572 (78.4878, 1.4754) -> (78.4878, 6.9754) construction
  arc A95 (60.4878, 6.9754) -> (58.4878, 4.9754) centre (60.4878, 4.9754) ccw
  line L573 (30, 2.2254) -> (30, 2.2254)
  arc A96 (30, 2.2254) -> (30.75, 1.4754) centre (30.75, 2.2254) ccw
  arc A97 (46, 4.9754) -> (44, 6.9754) centre (44, 4.9754) ccw
  line L574 (30.75, 1.4754) -> (21.25, 1.4754) construction
  line L575 (44, 2.9754) -> (30.75, 2.9754)
  arc A98 (30.75, 2.9754) -> (30, 2.2254) centre (30.75, 2.2254) ccw
  line L576 (46, 4.9754) -> (46, 4.9754)
  arc A99 (44, 2.9754) -> (46, 4.9754) centre (44, 4.9754) ccw
  line L577 (8, 6.9754) -> (44, 6.9754)
  arc A100 (21.25, 1.4754) -> (22, 2.2254) centre (21.25, 2.2254) ccw
  line L578 (21.25, 2.9754) -> (8, 2.9754)
  arc A101 (22, 2.2254) -> (21.25, 2.9754) centre (21.25, 2.2254) ccw
  line L579 (6, 4.9754) -> (6, 4.9754)
  arc A102 (6, 4.9754) -> (8, 2.9754) centre (8, 4.9754) ccw
  line L580 (22, 2.2254) -> (22, 2.2254)
  line L581 (26, 1.4754) -> (26, 6.9754) construction
  arc A103 (8, 6.9754) -> (6, 4.9754) centre (8, 4.9754) ccw
  line L582 (60.4878, -336.3489) -> (73.7378, -336.3489)
  line L583 (58.4878, -338.3489) -> (58.4878, -338.3489)
  arc A104 (60.4878, -336.3489) -> (58.4878, -338.3489) centre (60.4878, -338.3489) ccw
  arc A105 (58.4878, -338.3489) -> (60.4878, -340.3489) centre (60.4878, -338.3489) ccw
  line L584 (83.2378, -336.3489) -> (96.4878, -336.3489)
  line L585 (96.4878, -340.3489) -> (60.4878, -340.3489)
  line L586 (82.4878, -335.5989) -> (82.4878, -335.5989)
  arc A106 (82.4878, -335.5989) -> (83.2378, -336.3489) centre (83.2378, -335.5989) ccw
  arc A107 (83.2378, -334.8489) -> (82.4878, -335.5989) centre (83.2378, -335.5989) ccw
  line L587 (78.4878, -334.8489) -> (78.4878, -340.3489) construction
  line L588 (73.7378, -334.8489) -> (83.2378, -334.8489) construction
  line L589 (74.4878, -335.5989) -> (74.4878, -335.5989)
  arc A108 (74.4878, -335.5989) -> (73.7378, -334.8489) centre (73.7378, -335.5989) ccw
  arc A109 (73.7378, -336.3489) -> (74.4878, -335.5989) centre (73.7378, -335.5989) ccw
  arc A110 (98.4878, -338.3489) -> (96.4878, -336.3489) centre (96.4878, -338.3489) ccw
  arc A111 (96.4878, -340.3489) -> (98.4878, -338.3489) centre (96.4878, -338.3489) ccw
  line L590 (98.4878, -338.3489) -> (98.4878, -338.3489)
  line L591 (8, -336.3489) -> (21.25, -336.3489)
  line L592 (6, -338.3489) -> (6, -338.3489)
  arc A112 (8, -336.3489) -> (6, -338.3489) centre (8, -338.3489) ccw
  arc A113 (6, -338.3489) -> (8, -340.3489) centre (8, -338.3489) ccw
  line L593 (30.75, -336.3489) -> (44, -336.3489)
  line L594 (44, -340.3489) -> (8, -340.3489)
  line L595 (30, -335.5989) -> (30, -335.5989)
  arc A114 (30, -335.5989) -> (30.75, -336.3489) centre (30.75, -335.5989) ccw
  arc A115 (30.75, -334.8489) -> (30, -335.5989) centre (30.75, -335.5989) ccw
  line L596 (26, -334.8489) -> (26, -340.3489) construction
  line L597 (21.25, -334.8489) -> (30.75, -334.8489) construction
  line L598 (22, -335.5989) -> (22, -335.5989)
  arc A116 (22, -335.5989) -> (21.25, -334.8489) centre (21.25, -335.5989) ccw
  arc A117 (21.25, -336.3489) -> (22, -335.5989) centre (21.25, -335.5989) ccw
  arc A118 (46, -338.3489) -> (44, -336.3489) centre (44, -338.3489) ccw
  arc A119 (44, -340.3489) -> (46, -338.3489) centre (44, -338.3489) ccw
  line L599 (46, -338.3489) -> (46, -338.3489)
  point P0 (80.2132, -230.8369)
  point P1 (81.7132, -230.8369)
  point P2 (80.2132, -168.9225)
  point P3 (80.2132, -97.7732)
  point P4 (81.7132, -97.7732)
  point P5 (81.7132, -168.9225)
  point P6 (61.1632, -235.5992)
  point P7 (61.1632, -164.4499)
  point P8 (62.6632, -164.4499)
  point P9 (62.6632, -235.5992)
  point P10 (42.1132, -164.1614)
  point P11 (42.1132, -93.0121)
  point P12 (43.6132, -93.0121)
  point P13 (43.6132, -164.1614)
  point P14 (42.1132, -221.3109)
  point P15 (42.1132, -169.2119)
  point P16 (43.6132, -221.3109)
  point P17 (23.0632, -211.7859)
  point P18 (23.0632, -159.6869)
  point P19 (24.5632, -159.6869)
  point P20 (24.5632, -211.7859)
  point P21 (23.0632, -154.6359)
  point P22 (23.0632, -102.5369)
  point P23 (24.5632, -102.5369)
  point P24 (24.5632, -154.6359)
  point P25 (23.0632, -97.4861)
  point P26 (23.0632, -45.3871)
  point P27 (24.5632, -45.3871)
  point P28 (24.5632, -97.4861)
  point P29 (42.1132, -87.9611)
  point P30 (42.1132, -35.8621)
  point P31 (43.6132, -35.8621)
  point P32 (43.6132, -87.9611)
  point P33 (61.1632, -159.3989)
  point P34 (61.1632, -107.2999)
  point P35 (62.6632, -107.2999)
  point P36 (62.6632, -159.3989)
  point P37 (61.1632, -102.2489)
  point P38 (61.1632, -31.0996)
  point P39 (62.6632, -31.0996)
  point P40 (62.6632, -102.2489)
  point P41 (80.2132, -92.7239)
  point P42 (80.2132, -21.5746)
  point P43 (81.7132, -21.5746)
  point P44 (81.7132, -92.7239)
  point P45 (105.9878, -272.8489)
  point P46 (105.9878, -312.8489)
  point P47 (109.9878, -272.8489)
  point P48 (107.9878, -312.8489)
  point P49 (107.9878, -272.8489)
  point P50 (105.2378, -288.8489)
  point P51 (105.2378, -296.8489)
  point P52 (107.2378, -292.8489)
  point P53 (104.4878, -40.5246)
  point P54 (104.4878, -208.8489)
  point P55 (104.4878, -124.5246)
  point P56 (105.9878, -188.8489)
  point P57 (105.9878, -228.8489)
  point P58 (109.9878, -188.8489)
  point P59 (107.2378, -208.8489)
  point P60 (105.9878, -104.5246)
  point P61 (105.9878, -144.5246)
  point P62 (109.9878, -104.5246)
  point P63 (107.2378, -124.5246)
  point P64 (105.9878, -20.5246)
  point P65 (105.9878, -60.5246)
  point P66 (109.9878, -20.5246)
  point P67 (107.2378, -40.5246)
  point P68 (-1.5, -272.8489)
  point P69 (-1.5, -312.8489)
  point P70 (-5.5, -312.8489)
  point P71 (-2.75, -292.8489)
  point P72 (0, -292.8489)
  point P73 (0, -208.8489)
  point P74 (0, -124.5246)
  point P75 (0, -40.5246)
  point P76 (-5.5, -228.8489)
  point P77 (-1.5, -228.8489)
  point P78 (-2.75, -208.8489)
  point P79 (-1.5, -188.8489)
  point P80 (-5.5, -144.5246)
  point P81 (-1.5, -144.5246)
  point P82 (-2.75, -124.5246)
  point P83 (-1.5, -104.5246)
  point P84 (-5.5, -60.5246)
  point P85 (-1.5, -60.5246)
  point P86 (-2.75, -40.5246)
  point P87 (-1.5, -20.5246)
  point P88 (98.4878, 2.9754)
  point P89 (58.4878, 2.9754)
  point P90 (58.4878, 6.9754)
  point P91 (78.4878, 4.2254)
  point P92 (46, 2.9754)
  point P93 (6, 2.9754)
  point P94 (6, 6.9754)
  point P95 (26, 4.2254)
  point P96 (78.4878, -334.8489)
  point P97 (26, -334.8489)
  point P98 (58.4878, -336.3489)
  point P99 (78.4878, -337.5989)
  point P100 (98.4878, -336.3489)
  point P101 (98.4878, -340.3489)
  point P102 (78.4878, -334.8489)
  point P103 (6, -336.3489)
  point P104 (26, -337.5989)
  point P105 (46, -336.3489)
  point P106 (46, -340.3489)
  point P107 (26, -334.8489)
  point P108 (105.2378, -44.5246)
  point P109 (107.9878, -60.5246)
  point P110 (107.9878, -20.5246)
  point P111 (105.2378, -36.5246)
  point P112 (83.2378, 1.4754)
  point P113 (98.4878, 4.9754)
  point P114 (58.4878, 4.9754)
  point P115 (74.4878, 2.2254)
  point P116 (73.7378, 1.4754)
  point P117 (30.75, 1.4754)
  point P118 (30, 2.2254)
  point P119 (46, 4.9754)
  point P120 (6, 4.9754)
  point P121 (22, 2.2254)
  point P122 (21.25, 1.4754)
  point P123 (0, -35.7746)
  point P124 (-3.5, -20.5246)
  point P125 (-3.5, -60.5246)
  point P126 (0, -45.2746)
  point P127 (0, -119.7746)
  point P128 (-3.5, -104.5246)
  point P129 (-3.5, -144.5246)
  point P130 (0, -129.2746)
  point P131 (-3.5, -188.8489)
  point P132 (-3.5, -228.8489)
  point P133 (-3.5, -272.8489)
  point P134 (-3.5, -312.8489)
  point P135 (21.25, -334.8489)
  point P136 (22, -335.5989)
  point P137 (6, -338.3489)
  point P138 (46, -338.3489)
  point P139 (30, -335.5989)
  point P140 (30.75, -334.8489)
  point P141 (74.4878, -335.5989)
  point P142 (58.4878, -338.3489)
  point P143 (98.4878, -338.3489)
  point P144 (82.4878, -335.5989)
  point P145 (105.2378, -212.8489)
  point P146 (107.9878, -228.8489)
  point P147 (105.2378, -204.8489)
  point P148 (105.2378, -128.5246)
  point P149 (107.9878, -144.5246)
  point P150 (107.9878, -104.5246)
  point P151 (105.2378, -120.5246)
  dimension "d28" = 4
  dimension "d29" = 4
  dimension "d30" = 4
  dimension "d31" = 40
  dimension "d34" = 8
  dimension "d36" = 0.75
  dimension "d37" = 1.5
  dimension "d38" = 7
  dimension "d39" = 0.75
  dimension "d40" = 2
  dimension "d114" = 42
  dimension "d115" = 42
  dimension "d116" = 84
  dimension "d117" = 84
  dimension "d118" = 4
  dimension "d119" = 40
  dimension "d120" = 8
  dimension "d121" = 0.75
  dimension "d122" = 0.75
  dimension "d123" = 2
  dimension "d124" = 4
  dimension "d125" = 40
  dimension "d126" = 8
  dimension "d127" = 0.75
  dimension "d128" = 0.75
  dimension "d129" = 2
  dimension "d130" = 4
  dimension "d131" = 40
  dimension "d132" = 8
  dimension "d133" = 0.75
  dimension "d134" = 0.75
  dimension "d135" = 2
  dimension "d142" = 4
  dimension "d143" = 40
  dimension "d144" = 8
  dimension "d145" = 0.75
  dimension "d146" = 0.75
  dimension "d147" = 2
  dimension "d148" = 4
  dimension "d149" = 40
  dimension "d150" = 8
  dimension "d151" = 0.75
  dimension "d152" = 0.75
  dimension "d153" = 2
  dimension "d154" = 4
  dimension "d155" = 40
  dimension "d156" = 8
  dimension "d157" = 0.75
  dimension "d158" = 0.75
  dimension "d159" = 2
  dimension "d160" = 4
  dimension "d161" = 40
  dimension "d162" = 8
  dimension "d163" = 0.75